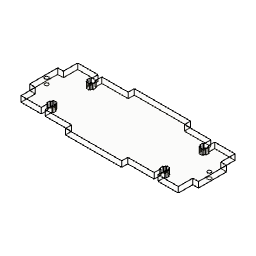
Carter_AvAr_KOSMOS3-0 (Autodesk Fusion 360 design; units mm, degrees)
Autodesk Fusion 360 part; units mm, degrees
sketch "Esquisse1" plane through (0, 0, 0) normal (0, 0, 1) x (1, 0, 0)
  line L0 (15.7988, 249.7948) -> (43.7076, 249.7948) construction
  line L1 (15.7988, 262.2639) -> (10.7166, 262.2639)
  line L2 (10.7166, 262.2639) -> (10.7166, 237.5139)
  line L3 (10.7166, 237.5139) -> (15.7988, 237.4198)
  line L4 (15.7988, 274.8948) -> (15.7988, 262.2639)
  line L5 (15.7988, 237.4198) -> (15.7988, 224.6948)
  line L6 (110.3988, 274.8948) -> (110.3988, 280.2948)
  line L7 (110.3988, 280.2948) -> (60.5988, 280.2948)
  line L8 (60.5988, 280.2948) -> (60.5988, 274.8948)
  line L9 (15.7988, 274.8948) -> (60.5988, 274.8948)
  line L10 (110.3988, 274.8948) -> (155.1988, 274.8948)
  line L11 (110.3988, 224.6948) -> (110.3988, 219.2948)
  line L12 (110.3988, 219.2948) -> (60.5988, 219.2948)
  line L13 (60.5988, 219.2948) -> (60.5988, 224.6948)
  line L14 (155.1988, 224.6948) -> (110.3988, 224.6948)
  line L15 (60.5988, 224.6948) -> (15.7988, 224.6948)
  line L16 (85.4988, 283.8421) -> (85.4988, 207.6137) construction
  line L17 (155.1988, 262.2639) -> (160.281, 262.2639)
  line L18 (160.281, 262.2639) -> (160.281, 237.5139)
  line L19 (160.281, 237.5139) -> (155.1988, 237.4198)
  line L20 (155.1988, 274.8948) -> (155.1988, 262.2639)
  line L21 (155.1988, 237.4198) -> (155.1988, 224.6948)
  circle A0 centre (13.4166, 249.7948) radius 1.6
  circle A1 centre (157.581, 249.7948) radius 1.6
  line L22 (33.7988, 274.8948) -> (37.1988, 274.8948)
  line L23 (37.1988, 274.8948) -> (37.1988, 268.8948)
  line L24 (33.7988, 268.8948) -> (33.7988, 274.8948)
  line L25 (35.4988, 277) -> (35.4988, 258) construction
  line L26 (32.7988, 268.8948) -> (32.7988, 266.1948)
  line L27 (38.1988, 266.1948) -> (38.1988, 268.8948)
  line L28 (37.1988, 266.1948) -> (37.1988, 264.6948)
  line L29 (36.6988, 264.1948) -> (34.2988, 264.1948)
  line L30 (33.7988, 264.6948) -> (33.7988, 266.1948)
  arc A2 (33.7988, 264.6948) -> (34.2988, 264.1948) centre (34.2988, 264.6948) ccw
  arc A3 (36.6988, 264.1948) -> (37.1988, 264.6948) centre (36.6988, 264.6948) ccw
  line L31 (32.7988, 266.1948) -> (33.7988, 266.1948)
  line L32 (37.1988, 266.1948) -> (38.1988, 266.1948)
  line L33 (38.1988, 268.8948) -> (37.1988, 268.8948)
  line L34 (33.7988, 268.8948) -> (32.7988, 268.8948)
  line L35 (33.7988, 234.8948) -> (33.7988, 233.3948)
  line L36 (37.1988, 233.3948) -> (38.1988, 233.3948)
  line L37 (38.1988, 233.3948) -> (38.1988, 230.6948)
  arc A4 (34.2988, 235.3948) -> (33.7988, 234.8948) centre (34.2988, 234.8948) ccw
  line L38 (32.7988, 230.6948) -> (32.7988, 233.3948)
  arc A5 (37.1988, 234.8948) -> (36.6988, 235.3948) centre (36.6988, 234.8948) ccw
  line L39 (36.6988, 235.3948) -> (34.2988, 235.3948)
  line L40 (37.1988, 233.3948) -> (37.1988, 234.8948)
  line L41 (32.7988, 233.3948) -> (33.7988, 233.3948)
  line L42 (33.7988, 230.6948) -> (32.7988, 230.6948)
  line L43 (38.1988, 230.6948) -> (37.1988, 230.6948)
  line L44 (33.7988, 230.6948) -> (33.7988, 224.6948)
  line L45 (37.1988, 224.6948) -> (37.1988, 230.6948)
  line L46 (138.1988, 268.8948) -> (138.1988, 266.1948)
  line L47 (137.1988, 230.6948) -> (138.1988, 230.6948)
  line L48 (133.7988, 233.3948) -> (133.7988, 234.8948)
  line L49 (132.7988, 268.8948) -> (133.7988, 268.8948)
  line L50 (138.1988, 233.3948) -> (137.1988, 233.3948)
  line L51 (132.7988, 266.1948) -> (132.7988, 268.8948)
  line L52 (133.7988, 266.1948) -> (133.7988, 264.6948)
  line L53 (133.7988, 266.1948) -> (132.7988, 266.1948)
  line L54 (132.7988, 233.3948) -> (132.7988, 230.6948)
  line L55 (137.1988, 268.8948) -> (138.1988, 268.8948)
  line L56 (137.1988, 234.8948) -> (137.1988, 233.3948)
  line L57 (138.1988, 230.6948) -> (138.1988, 233.3948)
  line L58 (134.2988, 264.1948) -> (136.6988, 264.1948)
  arc A6 (134.2988, 235.3948) -> (133.7988, 234.8948) centre (134.2988, 234.8948) ccw
  arc A7 (137.1988, 234.8948) -> (136.6988, 235.3948) centre (136.6988, 234.8948) ccw
  line L59 (132.7988, 230.6948) -> (133.7988, 230.6948)
  line L60 (138.1988, 266.1948) -> (137.1988, 266.1948)
  line L61 (137.1988, 264.6948) -> (137.1988, 266.1948)
  arc A8 (136.6988, 264.1948) -> (137.1988, 264.6948) centre (136.6988, 264.6948) ccw
  line L62 (134.2988, 235.3948) -> (136.6988, 235.3948)
  arc A9 (133.7988, 264.6948) -> (134.2988, 264.1948) centre (134.2988, 264.6948) ccw
  line L63 (133.7988, 233.3948) -> (132.7988, 233.3948)
  line L64 (137.1988, 230.6948) -> (137.1988, 224.6948)
  line L65 (133.7988, 224.6948) -> (133.7988, 230.6948)
  line L66 (137.1988, 268.8948) -> (137.1988, 274.8948)
  line L67 (133.7988, 274.8948) -> (133.7988, 268.8948)
  point P0 (155.1988, 249.7948)
  point P1 (33.7988, 264.1948)
  point P2 (33.7988, 235.3948)
  point P3 (127.2901, 249.7948)
  point P4 (137.1988, 235.3948)
  point P5 (135.4988, 258)
  point P6 (137.1988, 264.1948)
  dimension "d99" = 139.4
  dimension "d100" = 49.8
  dimension "d101" = 44.8
  dimension "d102" = 5.4
  dimension "d103" = 69.7
  dimension "d104" = 24.75
  dimension "d105" = 50.2
  dimension "d106" = 12.725
  dimension "d107" = 3.2
  dimension "d109" = 2.7
  dimension "d110" = 6
  dimension "d111" = 3.4
  dimension "d113" = 1.7
  dimension "d114" = 5.4
  dimension "d115" = 2.7
  dimension "d116" = 2.7
  dimension "d117" = 3.4
  dimension "d118" = 1.7
  dimension "d119" = 2
  dimension "d120" = 0.5
  dimension "d121" = 25.1
  constraint vertical L4
  constraint coincident L0.start L4
  constraint collinear L4 L5
  constraint perpendicular L4 L9
  constraint perpendicular L5 L14
  constraint vertical L6
  constraint horizontal L7
  constraint vertical L8
  constraint collinear L9 L10
  constraint symmetric L0 L8.end L13.end
  constraint symmetric L0 L6.start L11.start
  constraint symmetric L0 L6.end L11.end
  constraint symmetric L0 L7.end L12.end
  constraint collinear L14 L15
  constraint perpendicular L7 L16
  constraint symmetric L0.start L16 P0
  constraint symmetric L1.start L16 L17.start
  constraint symmetric L1.end L16 L17.end
  constraint symmetric L2.end L16 L18.end
  constraint symmetric L3.end L16 L19.end
  constraint collinear L20 L21
  constraint coincident L0 A0.centre
  constraint symmetric L16 A0 A1
  constraint horizontal L22
  constraint vertical L23
  constraint vertical L24
  constraint coincident L9 L22.start
  constraint horizontal L33
  constraint vertical L26
  constraint horizontal L31
  constraint vertical L27
  constraint vertical L28
  constraint horizontal L29
  constraint vertical L30
  constraint coincident P1 L29
  constraint coincident P1 L30
  constraint tangent L29 A2
  constraint tangent L30 A2
  constraint tangent L28 A3
  constraint tangent L29 A3
  constraint equal A2 A3
  constraint collinear L31 L32
  constraint collinear L33 L34
  constraint symmetric L0 L22.start L44.end
  constraint symmetric L0 L22.end L45.start
  constraint symmetric L0 L23.end L43.end
  constraint symmetric L0 L24.start L42.start
  constraint symmetric L0 L27.end L37.end
  constraint symmetric L0 L26.start L38.start
  constraint symmetric L0 L26.end L38.end
  constraint symmetric L0 L27.start L36.end
  constraint symmetric L0 L30.end L35.end
  constraint symmetric L0 L28.start L36.start
  constraint symmetric L0 P1 P2
  constraint symmetric L0 L29.end A4.start
  constraint symmetric L0 L30.start L35.start
  constraint symmetric L0 A2 A4
  constraint symmetric L0 L28.end A5.start
  constraint symmetric L0 L29.start A5.end
  constraint symmetric L0 A3 A5
  constraint symmetric L0.end L16 P3
  constraint symmetric L16 L22.start L66.end
  constraint symmetric L16 L22.end L67.start
  constraint symmetric L16 L23.end L49.end
  constraint symmetric L16 L24.start L55.start
  constraint symmetric L16 L25.end P5
  constraint symmetric L16 L27.end L49.start
  constraint symmetric L16 L26.start L46.start
  constraint symmetric L16 L26.end L46.end
  constraint symmetric L16 L27.start L51.start
  constraint symmetric L16 L30.end L60.end
  constraint symmetric L16 L28.start L52.start
  constraint symmetric L16 P1 P6
  constraint symmetric L16 L29.end L58.end
  constraint symmetric L16 L30.start L61.start
  constraint symmetric L16 A2 A8
  constraint symmetric L16 L28.end L52.end
  constraint symmetric L16 L29.start L58.start
  constraint symmetric L16 A3 A9
  constraint symmetric L16 L43.end L59.end
  constraint symmetric L16 A5.start L48.end
  constraint symmetric L16 P2 P4
  constraint symmetric L16 A5.end A6.start
  constraint symmetric L16 L36.end L54.start
  constraint symmetric L16 L38.end L50.start
  constraint symmetric L16 A4.start A7.end
  constraint symmetric L16 L38.start L47.end
  constraint symmetric L16 L36.start L48.start
  constraint symmetric L16 L37.end L54.end
  constraint symmetric L16 L35.start L56.start
  constraint symmetric L16 L42.start L47.start
  constraint symmetric L16 L35.end L50.end
  constraint symmetric L16 A4 A7
  constraint symmetric L16 A5 A6
  constraint symmetric L16 L44.end L64.end
  constraint symmetric L16 L45.start L65.start
  measures "d99" distance of L5.end L14.start
  measures "d100" distance of L6.end L7.end
  measures "d101" distance of L4.start L8.end
  measures "d102" distance of L8.end L7.end
  measures "d103" distance of L5 L16
  measures "d104" distance of L1.end L2.end
  measures "d105" distance of L4.start L5.end
  measures "d106" distance of L5.end L3.end
  measures "d107" diameter of A0
  measures "d109" distance of L2 A0.centre
  measures "d110" distance of L22.start L24.start
  measures "d111" distance of L23 L24
  measures "d113" distance of L24 L25
  measures "d114" distance of L26 L27
  measures "d115" distance of L26.start L26.end
  measures "d116" distance of L25 L27
  measures "d117" distance of L28 L30
  measures "d118" distance of L25 L30
  measures "d119" distance of L30.end P1
  measures "d120" radius of A2
  measures "d121" distance of L8 L25
extrude "Extrusion1" add sketch "Esquisse1" along normal blind 5 contours L1 L2 L3 L4 L5 L6 L7 L8 L9 L10 L11 L12 L13 L14 L15 L17 L18 L19 L20 L21 L23 L24 L26 L27 L28 L29 L30 A2 A3 L31 L32 L33 L34 L35 L36 L37 A4 L38 A5 L39 L40 L41 L42 L43 L44 L45 L46 L47 L48 L49 L50 L51 L52 L53 L54 L55 L56 L57 L58 A6 A7 L59 L60 L61 A8 L62 A9 L63 L64 L65 L66 L67
equation "d84 = 5.3 mm + 0.1 mm"
equation "d87 = 36 mm - 0.2 mm"
equation "d88 = 36 mm + 0.1 mm"
equation "d101 = ( d99 - d100 ) / 2"
equation "d103 = d99 / 2"
equation "d106 = ( d105 - d104 ) / 2"
equation "d109 = d102 / 2"
equation "d113 = d111 / 2"
equation "d116 = d114 / 2"
equation "d117 = d111"
equation "d118 = d117 / 2"
